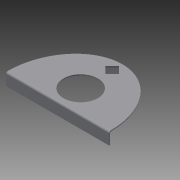
# Autodesk Inventor part: Patron
Saved by Autodesk Inventor 2015 SP1 (Build 190203100, 203)
## iProperties
Created: 2015-05-01
Part Number: Patron
Material: Générique
Document SubType Name: Modeling
Designer: Cyril
Density: 1 g/cm^3
Appearance: Par défaut
Author: Cyril
Autodesk Inventor part; units mm, degrees
ref_plane "YZ Plane" through (0, 0, 0) normal (1, 0, 0) x (0, 1, 0)
ref_plane "XZ Plane" through (0, 0, 0) normal (0, 1, 0) x (-1, 0, 0)
ref_plane "XY Plane" through (0, 0, 0) normal (0, 0, 1) x (1, 0, 0)
sketch "Sketch1" plane through (0, 0, 0) normal (0, 0, 1) x (1, 0, 0)
  arc A0 (105, 0) -> (-105, 0) centre (0, 0) ccw construction
  line L0 (0, -26) -> (0, 156) construction
  line L1 (-147, 0) -> (147, 0) construction
  line L2 (0, 123.2843) -> (14.1421, 109.1421)
  line L3 (14.1421, 109.1421) -> (0, 95)
  line L4 (0, 95) -> (-14.1421, 109.1421)
  line L5 (-14.1421, 109.1421) -> (0, 123.2843)
  line L6 (105, 0) -> (-105, 0)
  line L7 (-23, 45) -> (23, 45) construction
  circle A1 centre (0, 45) radius 35
  ellipse E0 centre (0, 0) end of major axis (0, -130) minor radius 105 (105, 0) -> (-105, 0) ccw
  line L8 (0, 0) -> (0, 130) construction
  dimension "d0" = 105
  dimension "d1" = 20
  dimension "d2" = 20
  dimension "d26" = 45
  dimension "d29" = 95
  dimension "d32" = 70
  dimension "d33" = 130
  constraints: 14 end point, 4 point on line, 2 centre point, 2 coincident, 2 parallel, 2 point on circle, 1 collinear, 1 horizontal, 1 midpoint, 1 perpendicular, 5 other
  measures "d0" radius of A0
  measures "d1" distance of L2.start L2.end
  measures "d2" distance of L4.end L2.start
  measures "d26" distance between parallel lines of L6 L7
  measures "d29" distance from line of L1 L3.end
  measures "d32" diameter of A1
  measures "d33" distance of L8.start L8.end
extrude "Extrusion3" add sketch "Sketch1" along normal blind 2
sketch "Sketch2" plane through (0, 0, 2) normal (0, 0, 1) x (1, 0, 0)
  line L0 (-105, 0) -> (105, 0)
  line L1 (105, 0) -> (105, -2)
  line L2 (105, -2) -> (-105, -2)
  line L3 (-105, -2) -> (-105, 0)
  ellipse E0 centre (0, 0) end of major axis (0, 130) minor radius 105 (105, 0) -> (-105, 0) ccw projected
  dimension "d36" = 2
  constraints: 8 end point, 2 parallel, 1 horizontal, 1 perpendicular, 1 other
  measures "d36" distance of L2.end L0.start
extrude "Extrusion4" add sketch "Sketch2" against normal blind 25 contours L0 L1 L2 L3
fillet "Fillet1" radius 4 1 edges at (0, -2, 2)
fillet "Fillet2" radius 2 1 edges at (0, 0, 0)
equation "\"d2\" = d1"
body "Solid3"
